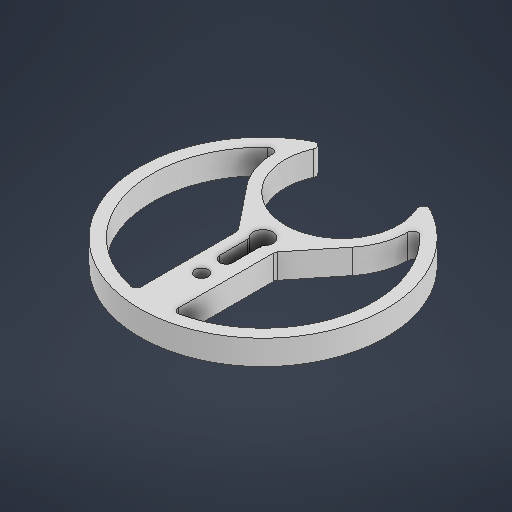
# Autodesk Inventor part: Gear Holder 1
Saved by Autodesk Inventor 2026.2 (Build 302298000, 298)
## iProperties
Created: 2026-01-26
Part Number: Gear Holder 1
Material: Generic
Document SubType Name: Modeling
Designer: Cobble
Density: 1 g/cm^3
Appearance: Default
Author: Cobble
Autodesk Inventor part; units mm, degrees
ref_plane "YZ Plane" through (0, 0, 0) normal (1, 0, 0) x (0, 1, 0)
ref_plane "XZ Plane" through (0, 0, 0) normal (0, 1, 0) x (-1, 0, 0)
ref_plane "XY Plane" through (0, 0, 0) normal (0, 0, 1) x (1, 0, 0)
sketch "Sketch1" plane through (0, 0, 0) normal (0, 0, 1) x (1, 0, 0)
  circle A0 centre (0, 0) radius 60.5521
  arc A1 (-0.7258, 10.3355) -> (0.2666, 10.325) centre (0, 32) ccw
  circle A2 centre (0, 0) radius 60.5521
  circle A3 centre (0, 32) radius 2.5
  circle A4 centre (0, 0) radius 50
  circle A5 centre (0, 0) radius 57.5
  circle A6 centre (0, 0) radius 57
  circle A7 centre (0, 0) radius 7.5
  circle A8 centre (0, 32) radius 23
  circle A9 centre (0, 0) radius 45
  circle A10 centre (0, 32) radius 27.5
  line L0 (-5.8547, -4.6875) -> (-21.4672, 14.8125)
  line L1 (5.8547, -4.6875) -> (21.4672, 14.8125)
  line L2 (0, 0) -> (0, 32)
  line L3 (7.5, 44.3706) -> (7.5, -44.3706)
  line L4 (-7.5, 44.3706) -> (-7.5, -44.3706)
  circle A11 centre (0, 0) radius 2.6
  line L5 (0, 0) -> (0, -15)
  circle A12 centre (0, -15) radius 2.6
  line L6 (-2.6, -15) -> (-2.6, 0)
  line L7 (2.6, 0) -> (2.6, -15)
  circle A13 centre (0, 0) radius 4
  line L8 (0, -15) -> (0, -25)
  circle A14 centre (0, -25) radius 2.6
  point P0 (27.2328, 35.8242)
  point P1 (7.5, -2.6325)
  point P2 (-27.2328, 35.8242)
  point P3 (-7.5, -2.6325)
  point P4 (17.6083, 46.7969)
  point P5 (-17.6083, 46.7969)
  point P6 (-2.6, -3.0397)
  point P7 (2.6, -3.0397)
  dimension "d0" = 5
  dimension "d1" = 100
  dimension "d2" = 115
  dimension "d4" = 15
  dimension "d5" = 46
  dimension "d6" = 90
  dimension "d7" = 55
  dimension "d8" = 32
  dimension "d12" = 5.2
  dimension "d13" = 15
  dimension "d14" = 5.2
  dimension "d15" = 8
  dimension "d17" = 10
  dimension "d18" = 5.2
  constraints: 18 end point, 15 centre point, 14 coincident, 14 point on circle, 9 tangent, 4 vertical, 2 parallel, 1 concentric
  measures "d0" diameter of A3
  measures "d1" diameter of A4
  measures "d2" diameter of A5
  measures "d4" diameter of A7
  measures "d5" diameter of A8
  measures "d6" diameter of A9
  measures "d7" diameter of A10
  measures "d8" distance of A1.centre A0.centre
  measures "d12" diameter of A11
  measures "d13" distance of L5.start L5.end
  measures "d14" diameter of A12
  measures "d15" diameter of A13
  measures "d17" distance of L8.start L8.end
  measures "d18" diameter of A14
extrude "Extrusion1" add sketch "Sketch1" along normal blind 10 contours A8 L3 A10 A7 L2 | L2 A7 A10 L4 A8 | L4 A10 A9 A8 | A8 A9 A10 L3 | L2 A10 A7 | A7 A10 L2 | A9 A10 A4 A8 | L4 L0 A10 | A10 A7 L4 | L3 A7 A10 | A10 L1 L3 | A7 L7 A13 L2 A10 | A10 L2 A13 L6 A7 | A9 A10 A4 | A7 L0 L4 | A8 A4 A10 A9 | L3 L1 A7 | L4 L0 A7 L6 A12 L7 L1 L3 A9
fillet "Fillet1" radius 2 8 edges at (-17.6083, 46.7969, 5) (17.6083, 46.7969, 5) (27.2328, 35.8242, 5) (-27.2328, 35.8242, 5) (-7.5, -2.6325, 5) (7.5, -2.6325, 5) (7.5, -44.3706, 5) (-7.5, -44.3706, 5)
fillet "Fillet2" radius 2 2 edges at (-2.6, -3.0397, 5) (2.6, -3.0397, 5)
body "Solid1"
